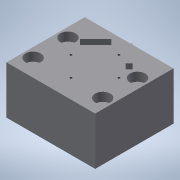
# Autodesk Inventor part: ResGalvoMount_base_plate
Saved by Autodesk Inventor 2022 (Build 260153000, 153)
## iProperties
Created: 2022-05-09
Part Number: ResGalvoMount_base_plate
Material: Generic
Document SubType Name: Modeling
Designer: kk4764
Density: 1 g/cm^3
Appearance: Default
Author: kk4764
Autodesk Inventor part; units mm, degrees
ref_plane "YZ Plane" through (0, 0, 0) normal (1, 0, 0) x (0, 1, 0)
ref_plane "XZ Plane" through (0, 0, 0) normal (0, 1, 0) x (-1, 0, 0)
ref_plane "XY Plane" through (0, 0, 0) normal (0, 0, 1) x (1, 0, 0)
sketch "Sketch1" plane through (0, 0, 0) normal (0, 1, 0) x (-1, 0, 0)
  line L0 (0, 0) -> (-64.77, 0)
  line L1 (-64.77, 0) -> (-64.77, -57.15)
  line L2 (-64.77, -57.15) -> (0, -57.15)
  line L3 (0, -57.15) -> (0, 0)
  dimension "d0" = 64.77
  dimension "d1" = 57.15
  constraints: 8 end point, 2 parallel, 1 horizontal, 1 perpendicular
  measures "d0" distance of L1.end L2.end
  measures "d1" distance of L0.end L1.end
extrude "Extrusion1" add sketch "Sketch1" along normal blind 34.9368
sketch "Sketch2" plane through (0, 34.9368, 0) normal (0, 1, 0) x (1, 0, 0)
  circle A0 centre (33.2953, 13.7711) radius 1.27
  line L0 (0, 0) -> (64.77, 0) projected
  line L1 (0, 57.15) -> (0, 0) projected
  circle A1 centre (18.8349, 28.2314) radius 1.27
  circle A2 centre (36.3358, 45.7323) radius 1.27
  line L2 (64.77, 57.15) -> (0, 57.15) projected
  circle A3 centre (50.7961, 31.2719) radius 1.27
  dimension "d4" = 13.7711
  dimension "d5" = 33.2953
  dimension "d6" = 2.54
  dimension "d7" = 2.54
  dimension "d8" = 28.2314
  dimension "d9" = 18.8349
  dimension "d10" = 2.54
  dimension "d11" = 11.4177
  dimension "d12" = 36.3358
  dimension "d13" = 2.54
  dimension "d14" = 25.8781
  dimension "d15" = 50.7961
  constraints: 4 centre point
  measures "d4" distance from line of L0 A0.centre
  measures "d5" distance from line of L1 A0.centre
  measures "d6" diameter of A0
  measures "d7" diameter of A1
  measures "d8" distance from line of L0 A1.centre
  measures "d9" distance from line of L1 A1.centre
  measures "d10" diameter of A2
  measures "d11" distance from line of L2 A2.centre
  measures "d12" distance from line of L1 A2.centre
  measures "d13" diameter of A3
  measures "d14" distance from line of L2 A3.centre
  measures "d15" distance from line of L1 A3.centre
hole "Hole1" at (50.7961, 34.9368, -31.2719) at (36.3358, 34.9368, -45.7323) at (18.8349, 34.9368, -28.2314) at (33.2953, 34.9368, -13.7711) direction (0, -1, 0) diameter 1.567 end through all thread size "M2x0.4" class "6H" standard "ANSI Metric M Profile"
sketch "Sketch3" plane through (0, 34.9368, 0) normal (0, 1, 0) x (1, 0, 0)
  circle A0 centre (6.8509, 12.5984) radius 1.27
  line L0 (0, 0) -> (64.77, 0) projected
  line L1 (0, 57.15) -> (0, 0) projected
  circle A1 centre (6.8509, 37.9984) radius 1.27
  circle A2 centre (57.6509, 37.9984) radius 1.27
  circle A3 centre (57.6509, 12.5984) radius 1.27
  dimension "d23" = 2.54
  dimension "d24" = 12.5984
  dimension "d25" = 6.8509
  dimension "d26" = 2.54
  dimension "d27" = 25.4
  dimension "d28" = 2.54
  dimension "d29" = 50.8
  dimension "d30" = 2.54
  dimension "d31" = 50.8
  constraints: 4 centre point
  measures "d23" diameter of A0
  measures "d24" distance from line of L0 A0.centre
  measures "d25" distance from line of L1 A0.centre
  measures "d26" diameter of A1
  measures "d27" distance of A0.centre A1.centre
  measures "d28" diameter of A2
  measures "d29" distance of A2.centre A1.centre
  measures "d30" diameter of A3
  measures "d31" distance of A0.centre A3.centre
hole "Hole2" at (57.6509, 34.9368, -37.9984) at (57.6509, 34.9368, -12.5984) at (6.8509, 34.9368, -12.5984) at (6.8509, 34.9368, -37.9984) direction (0, -1, 0) diameter 6.7564 end through all counterbore diameter 11.1252 counterbore depth 6.35 clearance for "Socket Head Cap Screw" size "1/4" standard "Ansi Unified Screw Threads"
sketch "Sketch4" plane through (0, 34.9368, 0) normal (0, 1, 0) x (1, 0, 0)
  line L0 (15.7866, 37.911) -> (27.2166, 49.341)
  line L1 (27.2166, 49.341) -> (24.6766, 51.881)
  line L2 (24.6766, 51.881) -> (13.2466, 40.451)
  line L3 (13.2466, 40.451) -> (15.7866, 37.911)
  line L4 (0, 57.15) -> (0, 0) projected
  dimension "d39" = 45
  dimension "d40" = 24.7669
  dimension "d41" = 2.54
  dimension "d42" = 11.43
  constraints: 8 end point, 2 perpendicular, 1 parallel
  measures "d39" angle of L4 L0
  measures "d40" distance from line of L4.start L0
  measures "d41" horizontal distance of L0.end L1.end
  measures "d42" horizontal distance of L1.end L2.end
extrude "Extrusion2" add sketch "Sketch4" along normal blind 3.81
sketch "Sketch5" plane through (0, 34.9368, 0) normal (0, 1, 0) x (1, 0, 0)
  line L0 (47.9873, 39.0305) -> (35.2873, 51.7305)
  line L1 (35.2873, 51.7305) -> (37.8273, 54.2705)
  line L2 (37.8273, 54.2705) -> (50.5273, 41.5705)
  line L3 (50.5273, 41.5705) -> (47.9873, 39.0305)
  line L4 (64.77, 0) -> (64.77, 57.15) projected
  point P0 (0, 0)
  dimension "d45" = 2.54
  dimension "d46" = 12.7
  dimension "d47" = 45
  dimension "d48" = 24.6795
  constraints: 8 end point, 3 perpendicular
  measures "d45" horizontal distance of L0.end L1.end
  measures "d46" horizontal distance of L1.end L2.end
  measures "d47" angle of L4 L2
  measures "d48" distance from line of L4.end L0
extrude "Extrusion3" add sketch "Sketch5" along normal blind 3.81
body "Solid1"
